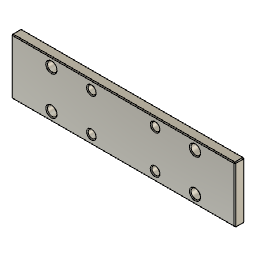
Z motor reinforcement plate (Autodesk Fusion 360 design; units mm, degrees)
Autodesk Fusion 360 part; units mm, degrees
sketch "Z motor reinforcement" plane through (0, 0, 0) normal (0, 1, 0) x (1, 0, 0)
  line L0 (-70, -17.4987) -> (70, -17.4987)
  circle A0 centre (-45, -11.9987) radius 3
  circle A1 centre (-45, 12.0013) radius 3
  circle A2 centre (45, -11.9987) radius 3
  circle A3 centre (45, 12.0013) radius 3
  circle A4 centre (20, -11.9799) radius 2.5
  line L1 (45, -13.5) -> (45, 16.5) construction
  line L2 (20, -13.5) -> (20, 16.5) construction
  line L3 (-54.8652, -11.9987) -> (55.1348, -11.9987) construction
  line L4 (70, 17.5013) -> (-70, 17.5013)
  line L5 (-45, -13.5) -> (-45, 16.5) construction
  line L6 (70, -17.4987) -> (70, 17.5013)
  line L7 (20, -11.9799) -> (20, 12) construction
  circle A5 centre (20, 12) radius 2.5
  line L8 (-55, 12.0013) -> (55, 12.0013) construction
  circle A6 centre (-20, 12) radius 2.5
  line L9 (-70, 17.5013) -> (-70, -17.4987)
  line L10 (-20, -11.985) -> (-20, 12) construction
  line L11 (-20, -13.5) -> (-20, 16.5) construction
  circle A7 centre (-20, -11.985) radius 2.5
  dimension "d1" = 140
  dimension "d2" = 35
  dimension "d3" = 110
  dimension "d4" = 24
  dimension "d5" = 25
  dimension "d6" = 40
  dimension "d7" = 25
  dimension "d8" = 25
  dimension "d9" = 6
  dimension "d10" = 6
  dimension "d11" = 6
  dimension "d12" = 6
  dimension "d13" = 5
  dimension "d14" = 5
  dimension "d15" = 5
  dimension "d16" = 5
  dimension "d17" = 5.5
  constraint horizontal L0
  constraint vertical L6
  constraint horizontal L4
  constraint vertical L9
  constraint parallel L0 L3
  constraint horizontal L8
  constraint perpendicular L5 L8
  constraint perpendicular L8 L11
  constraint perpendicular L2 L8
  constraint perpendicular L1 L8
  constraint coincident A0.centre L5
  constraint coincident A0.centre L3
  constraint coincident A1.centre L8
  constraint coincident A1.centre L5
  constraint coincident A2.centre L3
  constraint coincident A2.centre L1
  constraint coincident A3.centre L8
  constraint coincident A3.centre L1
  constraint coincident L10.start A7.centre
  constraint coincident A4.centre L7.start
  constraint coincident A6.centre L10.end
  constraint coincident L7.end A5.centre
  measures "d1" distance of L0.start L0.end
  measures "d2" distance of L4.end L0.start
  measures "d3" distance of L3.start L3.end
  measures "d4" distance of L3 L8
  measures "d5" distance of L5 L11
  measures "d6" distance of L2 L10
  measures "d7" distance of L1 L7
  measures "d8" distance of L1 L6
  measures "d9" diameter of A0
  measures "d10" diameter of A1
  measures "d11" diameter of A2
  measures "d12" diameter of A3
  measures "d13" diameter of A7
  measures "d14" diameter of A4
  measures "d15" diameter of A6
  measures "d16" diameter of A5
  measures "d17" distance of L0 L3
extrude "Extrude1" add sketch "Z motor reinforcement" along normal blind 6 makes body 1
copy_body "Body->Comp1" bodies 1 removing the originals makes body 2 in component "Z motor reinforcement"
chamfer "Chamfer1" distance 0.5 angle 45 27 edges at (0, 0, 17.4987) (-70, 3, 17.4987) (0, 6, 17.4987) (70, 3, 17.4987) (70, 6, -0.0013) (70, 0, -0.0013) (0, 0, -17.5013) (-70, 0, -0.0013) (-47.797, 0, 10.9138) (-47.797, 0, -13.0862) (-22.3308, 0, 11.081) (-22.3308, 0, -12.904) (17.6692, 0, 11.0759) (17.6692, 0, -12.904) (42.203, 0, 10.9138) (42.203, 0, -13.0862) (0, 6, -17.5013) (-70, 3, -17.5013) (-70, 6, -0.0013) (-47.797, 6, -13.0862) (-47.797, 6, 10.9138) (-22.3308, 6, 11.081) (17.6692, 6, 11.0759) (42.203, 6, 10.9138) (42.203, 6, -13.0862) (17.6692, 6, -12.904) (-22.3308, 6, -12.904) on bodies 2 in component "Z motor reinforcement"
component "Z motor reinforcement" placed x (1, 0, 0) y (0, 1, 0) z (0, 0, 1) at (0, 0, 0)
named bodies: "Plate"
